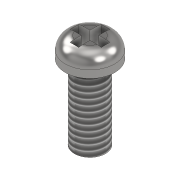
# Autodesk Inventor part: M4_8mm
Saved by Autodesk Inventor 2021 (Build 250183000, 183)
## iProperties
Created: 2022-06-08
Part Number: M4_8mm
Material: Stainless Steel
Document SubType Name: Modeling
Designer: alyn649
Density: 8 g/cm^3
Appearance: Semi-Polished
Author: alyn649
Autodesk Inventor part; units mm, degrees
ref_plane "YZ Plane" through (0, 0, 0) normal (1, 0, 0) x (0, 1, 0)
ref_plane "XZ Plane" through (0, 0, 0) normal (0, 1, 0) x (-1, 0, 0)
ref_plane "XY Plane" through (0, 0, 0) normal (0, 0, 1) x (1, 0, 0)
sketch "Sketch1" plane through (0, 0, 0) normal (0, 1, 0) x (-1, 0, 0)
  circle A0 centre (0, 0) radius 1.98
  dimension "d0" = 3.96
  constraints: 1 centre point, 1 coincident
  measures "d0" diameter of A0
extrude "Extrusion1" add sketch "Sketch1" along normal blind 1.6
sketch "Sketch2" plane through (0, 1.6, 0) normal (0, 1, 0) x (1, 0, 0)
  line L0 (-0.35, -0.35) -> (-1.25, -0.35)
  line L1 (-1.25, -0.35) -> (-1.25, 0.35)
  line L2 (-1.25, 0.35) -> (-0.35, 0.35)
  line L3 (-0.35, 0.35) -> (-0.35, 1.25)
  line L4 (-0.35, 1.25) -> (0.35, 1.25)
  line L5 (0.35, 1.25) -> (0.35, 0.35)
  line L6 (0.35, 0.35) -> (1.25, 0.35)
  line L7 (1.25, 0.35) -> (1.25, -0.35)
  line L8 (1.25, -0.35) -> (0.35, -0.35)
  line L9 (0.35, -1.25) -> (-0.35, -1.25)
  line L10 (-0.35, -1.25) -> (-0.35, -0.35)
  line L11 (0.35, -0.35) -> (0.35, -1.25)
  point P0 (0, 0)
  point P1 (0, -1.25)
  point P2 (0, 1.25)
  point P3 (-1.25, 0)
  point P4 (1.25, 0)
  dimension "d3" = 2.5
  dimension "d4" = 2.5
  dimension "d5" = 1.25
  dimension "d6" = 1.25
  dimension "d7" = 0.7
  dimension "d8" = 0.7
  constraints: 24 end point, 7 perpendicular, 7 point on line, 4 midpoint, 2 horizontal alignment, 2 parallel, 2 vertical alignment, 1 horizontal
  measures "d3" distance between parallel lines of L4 L9
  measures "d4" distance between parallel lines of L1 L7
  measures "d5" distance from line of point (0, 0) L7
  measures "d6" distance from line of point (0, 0) L4
  measures "d7" distance of L0.end L1.end
  measures "d8" distance of L9.start L9.end
extrude "Extrusion2" cut sketch "Sketch2" against normal blind 2
fillet "Fillet1" radius 1 1 edges at (1.98, 1.6, 0)
sketch "Sketch3" plane through (0, 0, 0) normal (0, -1, 0) x (1, 0, 0)
  circle A0 centre (0, 0) radius 1.25
  dimension "d12" = 2.5
  constraints: 1 centre point, 1 coincident
  measures "d12" diameter of A0
extrude "Extrusion3" add sketch "Sketch3" along normal blind 6
thread "Thread1" size "M2.5x0.45" class "6g" standard "ANSI Metric M Profile" full length
equation "\"d4\" = d3"
equation "\"d5\" = 0.5 * d4"
equation "\"d6\" = d5"
equation "\"d8\" = d7"
body "Solid1"
